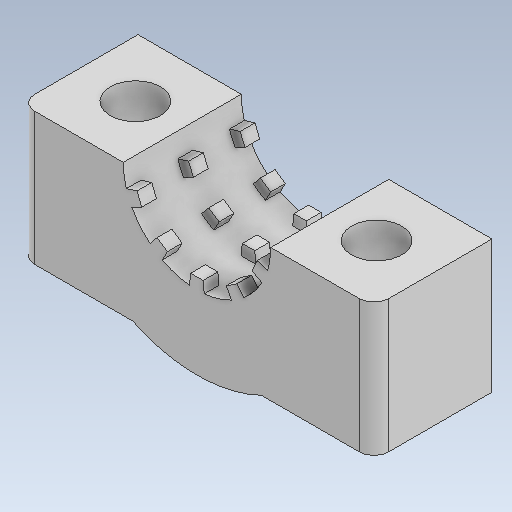
# Autodesk Inventor part: Bed Cable Harness Cable Clamp
Saved by Autodesk Inventor 2020.3 (Build 243373010, 373A)
## iProperties
Created: 2019-12-21
Part Number: Bed Cable Harness Cable Clamp
Material: Generic
Document SubType Name: Modeling
Designer: pepd9
Density: 1 g/cm^3
Appearance: Default
Author: pepd9
Autodesk Inventor part; units mm, degrees
ref_plane "YZ Plane" through (0, 0, 0) normal (1, 0, 0) x (0, 1, 0)
ref_plane "XZ Plane" through (0, 0, 0) normal (0, 1, 0) x (-1, 0, 0)
ref_plane "XY Plane" through (0, 0, 0) normal (0, 0, 1) x (1, 0, 0)
sketch "Sketch1" plane through (0, 0, 0) normal (0, 0, 1) x (1, 0, 0)
  arc A0 (5, -5) -> (-5, -5) centre (0, -5) ccw projected
  circle A1 centre (0, -5) radius 5
  arc A2 (4.3589, 4) -> (-4.3589, 4) centre (0, -5) ccw projected
  line L0 (12, -5) -> (12, 4) projected
  line L1 (11, 4) -> (4.3589, 4) projected
  line L2 (12, 4) -> (0, 4)
  line L3 (0, 4) -> (0, -5)
  line L4 (0, -5) -> (12, -5)
  line L5 (12, -5) -> (12, 4)
  arc A3 (-4.3589, -14) -> (4.3589, -14) centre (0, -5) ccw
  line L6 (12, -5) -> (12, -14)
  line L7 (12, -14) -> (0, -14)
  line L8 (-12, -5) -> (-12, 4)
  line L9 (-12, 4) -> (0, 4)
  line L10 (0, -5) -> (-12, -5)
  line L11 (-12, -14) -> (0, -14)
  line L12 (-12, -5) -> (-12, -14)
  circle A4 centre (0, -5) radius 10
  point P0 (0, 0)
  constraints: 22 end point, 8 symmetric about line, 2 coincident, 2 parallel, 2 point on circle, 1 centre point, 1 horizontal, 1 perpendicular, 7 other
ref_plane "Work Plane1" through (-11, -5, -8) normal (0, 0, -1) x (0, 1, 0)
extrude "Extrusion1" add sketch "Sketch1" against normal up to surface (8 mm away) contours L4 A4 L7 L11 L10 A1 | L4 L6 L7 A4 | A4 L11 L12 L10 | A3 L11 L7
sketch "Sketch2" plane through (4.3589, -14, 0) normal (0, -1, 0) x (1, 0, 0)
  circle A0 centre (3.8206, -4) radius 1.7 projected
  circle A1 centre (-12.5383, -4) radius 1.7 projected
  point P0 (-4.3589, 0)
hole "Hole1" at (-8.1794, -14, -4) at (8.1794, -14, -4) direction (0, 1, 0) diameter 3.4 end through all counterbore diameter 6.5 counterbore depth 3 clearance for "Socket Head Cap Screw" size "M3" standard "Ansi Metric M Profile"
fillet "Fillet1" radius 1 2 edges at (12, -9.5, 0) (-12, -9.5, 0)
sketch "Sketch3" plane through (0, 0, 0) normal (0, 0, 1) x (1, 0, 0)
  line L0 (-8, 4.75) -> (11, 4.75) projected
  line L1 (-8, 4.75) -> (-8, -5) projected
  line L2 (-8, -5) -> (-5, -5) projected
  arc A0 (-4.7896, -3.5647) -> (-5, -5) centre (0, -5) ccw projected
  line L3 (-4.7896, -3.5647) -> (-4.0711, -3.78) projected
  line L4 (-4.0711, -3.78) -> (-3.7492, -2.9985) projected
  line L5 (-3.7492, -2.9985) -> (-4.4108, -2.6453) projected
  arc A1 (-3.185, -1.1457) -> (-4.4108, -2.6453) centre (0, -5) ccw projected
  line L6 (-3.185, -1.1457) -> (-2.7072, -1.7238) projected
  line L7 (-2.7072, -1.7238) -> (-2.0054, -1.2529) projected
  line L8 (-2.0054, -1.2529) -> (-2.3593, -0.5916) projected
  arc A2 (-0.5069, -0.0258) -> (-2.3593, -0.5916) centre (0, -5) ccw projected
  line L9 (-0.5069, -0.0258) -> (-0.4308, -0.7719) projected
  line L10 (-0.4308, -0.7719) -> (0.4144, -0.7702) projected
  line L11 (0.4144, -0.7702) -> (0.4875, -0.0238) projected
  arc A3 (2.3421, -0.5825) -> (0.4875, -0.0238) centre (0, -5) ccw projected
  line L12 (2.3421, -0.5825) -> (1.9908, -1.2451) projected
  line L13 (1.9908, -1.2451) -> (2.6945, -1.7133) projected
  line L14 (2.6945, -1.7133) -> (3.17, -1.1333) projected
  arc A4 (4.4016, -2.6282) -> (3.17, -1.1333) centre (0, -5) ccw projected
  line L15 (4.4016, -2.6282) -> (3.7414, -2.9839) projected
  line L16 (3.7414, -2.9839) -> (4.0664, -3.7642) projected
  line L17 (4.0664, -3.7642) -> (4.7839, -3.5461) projected
  arc A5 (5, -5) -> (4.7839, -3.5461) centre (0, -5) ccw projected
  line L18 (5, -5) -> (11, -5) projected
  line L19 (11, 4.75) -> (11, -5) projected
  circle A6 centre (0, -5) radius 5
  line L20 (-4.7896, -6.4353) -> (-4.0711, -6.22)
  line L21 (-4.0711, -6.22) -> (-3.7492, -7.0015)
  line L22 (-3.7492, -7.0015) -> (-4.4108, -7.3547)
  arc A7 (-4.4108, -7.3547) -> (-3.185, -8.8543) centre (0, -5) ccw
  line L23 (-3.185, -8.8543) -> (-2.7072, -8.2762)
  line L24 (-2.7072, -8.2762) -> (-2.0054, -8.7471)
  line L25 (-2.0054, -8.7471) -> (-2.3593, -9.4084)
  arc A8 (-2.3593, -9.4084) -> (-0.5069, -9.9742) centre (0, -5) ccw
  line L26 (-0.5069, -9.9742) -> (-0.4308, -9.2281)
  line L27 (-0.4308, -9.2281) -> (0.4144, -9.2298)
  line L28 (0.4144, -9.2298) -> (0.4875, -9.9762)
  arc A9 (0.4875, -9.9762) -> (2.3421, -9.4175) centre (0, -5) ccw
  line L29 (2.3421, -9.4175) -> (1.9908, -8.7549)
  line L30 (1.9908, -8.7549) -> (2.6945, -8.2867)
  line L31 (2.6945, -8.2867) -> (3.17, -8.8667)
  arc A10 (3.17, -8.8667) -> (4.4016, -7.3718) centre (0, -5) ccw
  line L32 (4.4016, -7.3718) -> (3.7414, -7.0161)
  line L33 (3.7414, -7.0161) -> (4.0664, -6.2358)
  line L34 (4.0664, -6.2358) -> (4.7839, -6.4539)
  point P0 (0, 0)
  point P1 (0, -10)
  point P2 (-4.4108, -7.3547)
  point P3 (-0.5069, -9.9742)
  point P4 (2.3421, -9.4175)
  point P5 (4.4016, -7.3718)
  constraints: 30 end point, 21 symmetric about line, 8 point on circle, 4 centre point, 1 coincident, 7 other
extrude "Extrusion2" add sketch "Sketch3" against normal blind 1 contours L20 L21 L22 A6 | A6 L32 L33 L34 | L23 L24 L25 A6 | A6 L29 L30 L31 | L26 L27 L28 A6
pattern_linear "Rectangular Pattern1" count 3 spacing 3.5 along (0, 0, -1) of "Extrusion2"
body "Solid1"
